Autodesk Fusion 360 part; units mm, degrees
(part 6 of 12)
  arc A2269 (96.3654, -39.4411) -> (96.0604, -39.4411) centre (96.2129, -39.4411) ccw
  arc A2270 (150.9862, -40.1688) -> (151.2912, -40.1688) centre (151.1387, -40.1688) ccw
  arc A2271 (151.2912, -40.1688) -> (150.9862, -40.1688) centre (151.1387, -40.1688) ccw
  arc A2272 (44.7289, -41.9748) -> (45.0339, -41.9748) centre (44.8814, -41.9748) ccw
  arc A2273 (45.0339, -41.9748) -> (44.7289, -41.9748) centre (44.8814, -41.9748) ccw
  arc A2274 (163.9811, 37.8053) -> (164.2861, 37.8053) centre (164.1336, 37.8053) ccw
  arc A2275 (164.2861, 37.8053) -> (163.9811, 37.8053) centre (164.1336, 37.8053) ccw
  arc A2276 (146.0527, -13.2374) -> (146.3577, -13.2374) centre (146.2052, -13.2374) ccw
  arc A2277 (146.3577, -13.2374) -> (146.0527, -13.2374) centre (146.2052, -13.2374) ccw
  arc A2278 (176.4441, -9.8328) -> (176.7491, -9.8328) centre (176.5966, -9.8328) ccw
  arc A2279 (176.7491, -9.8328) -> (176.4441, -9.8328) centre (176.5966, -9.8328) ccw
  arc A2280 (116.1959, -12.0024) -> (115.8909, -12.0024) centre (116.0434, -12.0024) ccw
  arc A2281 (115.8909, -12.0024) -> (116.1959, -12.0024) centre (116.0434, -12.0024) ccw
  arc A2282 (150.7728, -10.1653) -> (150.4678, -10.1653) centre (150.6203, -10.1653) ccw
  arc A2283 (150.4678, -10.1653) -> (150.7728, -10.1653) centre (150.6203, -10.1653) ccw
  arc A2284 (85.9928, -12.5211) -> (86.2978, -12.5211) centre (86.1453, -12.5211) ccw
  arc A2285 (86.2978, -12.5211) -> (85.9928, -12.5211) centre (86.1453, -12.5211) ccw
  arc A2286 (116.6014, -9.5793) -> (116.9064, -9.5793) centre (116.7539, -9.5793) ccw
  arc A2287 (116.9064, -9.5793) -> (116.6014, -9.5793) centre (116.7539, -9.5793) ccw
  arc A2288 (43.8853, -19.9798) -> (44.1903, -19.9798) centre (44.0378, -19.9798) ccw
  arc A2289 (44.1903, -19.9798) -> (43.8853, -19.9798) centre (44.0378, -19.9798) ccw
  arc A2290 (91.0235, -13.194) -> (91.3285, -13.194) centre (91.176, -13.194) ccw
  arc A2291 (91.3285, -13.194) -> (91.0235, -13.194) centre (91.176, -13.194) ccw
  arc A2292 (217.3525, -62.0055) -> (217.6575, -62.0055) centre (217.505, -62.0055) ccw
  arc A2293 (217.6575, -62.0055) -> (217.3525, -62.0055) centre (217.505, -62.0055) ccw
  arc A2294 (186.1886, -6.5094) -> (185.8836, -6.5094) centre (186.0361, -6.5094) ccw
  arc A2295 (185.8836, -6.5094) -> (186.1886, -6.5094) centre (186.0361, -6.5094) ccw
  arc A2296 (150.3339, -28.8564) -> (150.6389, -28.8564) centre (150.4864, -28.8564) ccw
  arc A2297 (150.6389, -28.8564) -> (150.3339, -28.8564) centre (150.4864, -28.8564) ccw
  arc A2298 (145.1401, -60.2572) -> (145.4451, -60.2572) centre (145.2926, -60.2572) ccw
  arc A2299 (145.4451, -60.2572) -> (145.1401, -60.2572) centre (145.2926, -60.2572) ccw
  arc A2300 (119.5917, -66.7802) -> (119.8967, -66.7802) centre (119.7442, -66.7802) ccw
  arc A2301 (119.8967, -66.7802) -> (119.5917, -66.7802) centre (119.7442, -66.7802) ccw
  arc A2302 (168.2221, 11.5998) -> (168.5272, 11.5998) centre (168.3747, 11.5998) ccw
  arc A2303 (168.5272, 11.5998) -> (168.2221, 11.5998) centre (168.3747, 11.5998) ccw
  arc A2304 (194.7456, 20.9148) -> (195.0506, 20.9148) centre (194.8981, 20.9148) ccw
  arc A2305 (195.0506, 20.9148) -> (194.7456, 20.9148) centre (194.8981, 20.9148) ccw
  arc A2306 (99.0245, 26.218) -> (99.3295, 26.218) centre (99.177, 26.218) ccw
  arc A2307 (99.3295, 26.218) -> (99.0245, 26.218) centre (99.177, 26.218) ccw
  arc A2308 (70.4291, -16.6778) -> (70.1241, -16.6778) centre (70.2766, -16.6778) ccw
  arc A2309 (70.1241, -16.6778) -> (70.4291, -16.6778) centre (70.2766, -16.6778) ccw
  arc A2310 (134.9499, 16.8688) -> (135.2549, 16.8688) centre (135.1024, 16.8688) ccw
  arc A2311 (135.2549, 16.8688) -> (134.9499, 16.8688) centre (135.1024, 16.8688) ccw
  arc A2312 (165.5168, 20.1454) -> (165.8218, 20.1454) centre (165.6693, 20.1454) ccw
  arc A2313 (165.8218, 20.1454) -> (165.5168, 20.1454) centre (165.6693, 20.1454) ccw
  arc A2314 (100.893, 26.9607) -> (101.198, 26.9607) centre (101.0455, 26.9607) ccw
  arc A2315 (101.198, 26.9607) -> (100.893, 26.9607) centre (101.0455, 26.9607) ccw
  arc A2316 (86.6801, -6.1922) -> (86.9851, -6.1922) centre (86.8326, -6.1922) ccw
  arc A2317 (86.9851, -6.1922) -> (86.6801, -6.1922) centre (86.8326, -6.1922) ccw
  arc A2318 (104.3532, 16.8617) -> (104.6582, 16.8617) centre (104.5057, 16.8617) ccw
  arc A2319 (104.6582, 16.8617) -> (104.3532, 16.8617) centre (104.5057, 16.8617) ccw
  arc A2320 (124.5234, 15.4924) -> (124.8284, 15.4924) centre (124.6759, 15.4924) ccw
  arc A2321 (124.8284, 15.4924) -> (124.5234, 15.4924) centre (124.6759, 15.4924) ccw
  arc A2322 (20.8272, 14.645) -> (21.1322, 14.645) centre (20.9797, 14.645) ccw
  arc A2323 (21.1322, 14.645) -> (20.8272, 14.645) centre (20.9797, 14.645) ccw
  arc A2324 (21.2366, 18.769) -> (21.5416, 18.769) centre (21.3891, 18.769) ccw
  arc A2325 (21.5416, 18.769) -> (21.2366, 18.769) centre (21.3891, 18.769) ccw
  arc A2326 (38.9043, 16.8274) -> (38.5993, 16.8274) centre (38.7518, 16.8274) ccw
  arc A2327 (38.5993, 16.8274) -> (38.9043, 16.8274) centre (38.7518, 16.8274) ccw
  arc A2328 (75.6966, 20.0435) -> (76.0016, 20.0435) centre (75.8491, 20.0435) ccw
  arc A2329 (76.0016, 20.0435) -> (75.6966, 20.0435) centre (75.8491, 20.0435) ccw
  arc A2330 (216.5973, 36.5028) -> (216.9023, 36.5028) centre (216.7498, 36.5028) ccw
  arc A2331 (216.9023, 36.5028) -> (216.5973, 36.5028) centre (216.7498, 36.5028) ccw
  arc A2332 (62.4485, 36.5028) -> (62.7535, 36.5028) centre (62.601, 36.5028) ccw
  arc A2333 (62.7535, 36.5028) -> (62.4485, 36.5028) centre (62.601, 36.5028) ccw
  arc A2334 (124.4947, 49.6851) -> (124.7997, 49.6851) centre (124.6472, 49.6851) ccw
  arc A2335 (124.7997, 49.6851) -> (124.4947, 49.6851) centre (124.6472, 49.6851) ccw
  arc A2336 (92.9478, -27.5572) -> (93.2528, -27.5572) centre (93.1003, -27.5572) ccw
  arc A2337 (93.2528, -27.5572) -> (92.9478, -27.5572) centre (93.1003, -27.5572) ccw
  arc A2338 (158.911, 44.4614) -> (159.216, 44.4614) centre (159.0635, 44.4614) ccw
  arc A2339 (159.216, 44.4614) -> (158.911, 44.4614) centre (159.0635, 44.4614) ccw
  arc A2340 (184.7538, 44.4614) -> (185.0588, 44.4614) centre (184.9063, 44.4614) ccw
  arc A2341 (185.0588, 44.4614) -> (184.7538, 44.4614) centre (184.9063, 44.4614) ccw
  arc A2342 (118.6672, 12.5444) -> (118.9722, 12.5444) centre (118.8197, 12.5444) ccw
  arc A2343 (118.9722, 12.5444) -> (118.6672, 12.5444) centre (118.8197, 12.5444) ccw
  arc A2344 (127.2216, 57.1512) -> (127.5266, 57.1512) centre (127.3741, 57.1512) ccw
  arc A2345 (127.5266, 57.1512) -> (127.2216, 57.1512) centre (127.3741, 57.1512) ccw
  arc A2346 (128.9905, 44.4614) -> (129.2955, 44.4614) centre (129.143, 44.4614) ccw
  arc A2347 (129.2955, 44.4614) -> (128.9905, 44.4614) centre (129.143, 44.4614) ccw
  arc A2348 (159.434, 50.1576) -> (159.739, 50.1576) centre (159.5865, 50.1576) ccw
  arc A2349 (159.739, 50.1576) -> (159.434, 50.1576) centre (159.5865, 50.1576) ccw
  arc A2350 (98.9415, 44.4614) -> (99.2465, 44.4614) centre (99.094, 44.4614) ccw
  arc A2351 (99.2465, 44.4614) -> (98.9415, 44.4614) centre (99.094, 44.4614) ccw
  arc A2352 (106.8124, 44.4614) -> (107.1174, 44.4614) centre (106.9649, 44.4614) ccw
  arc A2353 (107.1174, 44.4614) -> (106.8124, 44.4614) centre (106.9649, 44.4614) ccw
  arc A2354 (112.9504, 50.5993) -> (113.2554, 50.5993) centre (113.1029, 50.5993) ccw
  arc A2355 (113.2554, 50.5993) -> (112.9504, 50.5993) centre (113.1029, 50.5993) ccw
  arc A2356 (129.2079, 50.5993) -> (129.5129, 50.5993) centre (129.3604, 50.5993) ccw
  arc A2357 (129.5129, 50.5993) -> (129.2079, 50.5993) centre (129.3604, 50.5993) ccw
  arc A2358 (68.8676, 44.4614) -> (69.1726, 44.4614) centre (69.0201, 44.4614) ccw
  arc A2359 (69.1726, 44.4614) -> (68.8676, 44.4614) centre (69.0201, 44.4614) ccw
  arc A2360 (99.6842, 49.9803) -> (99.9892, 49.9803) centre (99.8367, 49.9803) ccw
  arc A2361 (99.9892, 49.9803) -> (99.6842, 49.9803) centre (99.8367, 49.9803) ccw
  arc A2362 (51.0316, 50.5033) -> (51.3367, 50.5033) centre (51.1842, 50.5033) ccw
  arc A2363 (51.3367, 50.5033) -> (51.0316, 50.5033) centre (51.1842, 50.5033) ccw
  arc A2364 (73.5005, 49.883) -> (73.8055, 49.883) centre (73.653, 49.883) ccw
  arc A2365 (73.8055, 49.883) -> (73.5005, 49.883) centre (73.653, 49.883) ccw
  arc A2366 (221.1025, -27.0019) -> (221.4075, -27.0019) centre (221.255, -27.0019) ccw
  arc A2367 (221.4075, -27.0019) -> (221.1025, -27.0019) centre (221.255, -27.0019) ccw
  arc A2368 (218.1536, 60.5599) -> (218.4586, 60.5599) centre (218.3061, 60.5599) ccw
  arc A2369 (218.4586, 60.5599) -> (218.1536, 60.5599) centre (218.3061, 60.5599) ccw
  arc A2370 (43.6496, 60.5599) -> (43.9546, 60.5599) centre (43.8021, 60.5599) ccw
  arc A2371 (43.9546, 60.5599) -> (43.6496, 60.5599) centre (43.8021, 60.5599) ccw
  arc A2372 (188.8485, 74.8421) -> (189.1535, 74.8421) centre (189.001, 74.8421) ccw
  arc A2373 (189.1535, 74.8421) -> (188.8485, 74.8421) centre (189.001, 74.8421) ccw
  arc A2374 (200.9369, 74.8421) -> (201.2419, 74.8421) centre (201.0894, 74.8421) ccw
  arc A2375 (201.2419, 74.8421) -> (200.9369, 74.8421) centre (201.0894, 74.8421) ccw
  arc A2376 (95.5287, 66.3102) -> (95.2237, 66.3102) centre (95.3762, 66.3102) ccw
  arc A2377 (95.2237, 66.3102) -> (95.5287, 66.3102) centre (95.3762, 66.3102) ccw
  arc A2378 (63.9466, -23.0278) -> (64.2516, -23.0278) centre (64.0991, -23.0278) ccw
  arc A2379 (64.2516, -23.0278) -> (63.9466, -23.0278) centre (64.0991, -23.0278) ccw
  arc A2380 (92.0195, -20.5656) -> (92.3245, -20.5656) centre (92.172, -20.5656) ccw
  arc A2381 (92.3245, -20.5656) -> (92.0195, -20.5656) centre (92.172, -20.5656) ccw
  arc A2382 (65.5109, 83.9028) -> (65.816, 83.9028) centre (65.6634, 83.9028) ccw
  arc A2383 (65.816, 83.9028) -> (65.5109, 83.9028) centre (65.6634, 83.9028) ccw
  arc A2384 (35.4591, -9.865) -> (35.7641, -9.865) centre (35.6116, -9.865) ccw
  arc A2385 (35.7641, -9.865) -> (35.4591, -9.865) centre (35.6116, -9.865) ccw
  arc A2386 (35.4568, -3.5704) -> (35.7618, -3.5704) centre (35.6093, -3.5704) ccw
  arc A2387 (35.7618, -3.5704) -> (35.4568, -3.5704) centre (35.6093, -3.5704) ccw
  arc A2388 (69.1045, 74.231) -> (69.4096, 74.231) centre (69.257, 74.231) ccw
  arc A2389 (69.4096, 74.231) -> (69.1045, 74.231) centre (69.257, 74.231) ccw
  arc A2390 (104.9132, 74.231) -> (104.6082, 74.231) centre (104.7607, 74.231) ccw
  arc A2391 (104.6082, 74.231) -> (104.9132, 74.231) centre (104.7607, 74.231) ccw
  arc A2392 (18.7687, -49.6804) -> (18.4637, -49.6804) centre (18.6162, -49.6804) ccw
  arc A2393 (18.4637, -49.6804) -> (18.7687, -49.6804) centre (18.6162, -49.6804) ccw
  arc A2394 (22.6862, -60.4264) -> (22.3812, -60.4264) centre (22.5337, -60.4264) ccw
  arc A2395 (22.3812, -60.4264) -> (22.6862, -60.4264) centre (22.5337, -60.4264) ccw
  arc A2396 (142.6481, 77.1248) -> (142.3431, 77.1248) centre (142.4956, 77.1248) ccw
  arc A2397 (142.3431, 77.1248) -> (142.6481, 77.1248) centre (142.4956, 77.1248) ccw
  arc A2398 (134.7352, 77.1248) -> (134.4302, 77.1248) centre (134.5827, 77.1248) ccw
  arc A2399 (134.4302, 77.1248) -> (134.7352, 77.1248) centre (134.5827, 77.1248) ccw
  arc A2400 (155.7745, 57.7646) -> (155.4695, 57.7646) centre (155.622, 57.7646) ccw
  arc A2401 (155.4695, 57.7646) -> (155.7745, 57.7646) centre (155.622, 57.7646) ccw
  arc A2402 (159.8904, 57.7646) -> (159.5854, 57.7646) centre (159.7379, 57.7646) ccw
  arc A2403 (159.5854, 57.7646) -> (159.8904, 57.7646) centre (159.7379, 57.7646) ccw
  arc A2404 (5.7362, 29.8711) -> (5.4312, 29.8711) centre (5.5837, 29.8711) ccw
  arc A2405 (5.4312, 29.8711) -> (5.7362, 29.8711) centre (5.5837, 29.8711) ccw
  arc A2406 (13.8419, -37.0289) -> (13.5369, -37.0289) centre (13.6894, -37.0289) ccw
  arc A2407 (13.5369, -37.0289) -> (13.8419, -37.0289) centre (13.6894, -37.0289) ccw
  arc A2408 (13.0738, -57.8284) -> (12.7688, -57.8284) centre (12.9213, -57.8284) ccw
  arc A2409 (12.7688, -57.8284) -> (13.0738, -57.8284) centre (12.9213, -57.8284) ccw
  arc A2410 (16.8027, -57.3339) -> (16.4977, -57.3339) centre (16.6502, -57.3339) ccw
  arc A2411 (16.4977, -57.3339) -> (16.8027, -57.3339) centre (16.6502, -57.3339) ccw
  arc A2412 (10.6361, 67.0153) -> (10.3311, 67.0153) centre (10.4836, 67.0153) ccw
  arc A2413 (10.3311, 67.0153) -> (10.6361, 67.0153) centre (10.4836, 67.0153) ccw
  arc A2414 (14.7771, 16.4842) -> (14.4721, 16.4842) centre (14.6246, 16.4842) ccw
  arc A2415 (14.4721, 16.4842) -> (14.7771, 16.4842) centre (14.6246, 16.4842) ccw
  arc A2416 (23.579, 16.4842) -> (23.274, 16.4842) centre (23.4265, 16.4842) ccw
  arc A2417 (23.274, 16.4842) -> (23.579, 16.4842) centre (23.4265, 16.4842) ccw
  arc A2418 (17.122, -56.3786) -> (16.817, -56.3786) centre (16.9695, -56.3786) ccw
  arc A2419 (16.817, -56.3786) -> (17.122, -56.3786) centre (16.9695, -56.3786) ccw
  arc A2420 (15.17, -53.6621) -> (14.865, -53.6621) centre (15.0175, -53.6621) ccw
  arc A2421 (14.865, -53.6621) -> (15.17, -53.6621) centre (15.0175, -53.6621) ccw
  arc A2422 (16.2236, -61.0169) -> (15.9186, -61.0169) centre (16.0711, -61.0169) ccw
  arc A2423 (15.9186, -61.0169) -> (16.2236, -61.0169) centre (16.0711, -61.0169) ccw
  arc A2424 (161.3656, -5.432) -> (161.0606, -5.432) centre (161.2131, -5.432) ccw
  arc A2425 (161.0606, -5.432) -> (161.3656, -5.432) centre (161.2131, -5.432) ccw
  arc A2426 (41.9593, -4.8617) -> (42.2643, -4.8617) centre (42.1118, -4.8617) ccw
  arc A2427 (42.2643, -4.8617) -> (41.9593, -4.8617) centre (42.1118, -4.8617) ccw
  arc A2428 (217.7147, 48.9513) -> (218.0197, 48.9513) centre (217.8672, 48.9513) ccw
  arc A2429 (218.0197, 48.9513) -> (217.7147, 48.9513) centre (217.8672, 48.9513) ccw
  arc A2430 (192.6885, -2.8919) -> (192.9935, -2.8919) centre (192.841, -2.8919) ccw
  arc A2431 (192.9935, -2.8919) -> (192.6885, -2.8919) centre (192.841, -2.8919) ccw
  arc A2432 (208.6974, 31.9866) -> (209.0024, 31.9866) centre (208.8499, 31.9866) ccw
  arc A2433 (209.0024, 31.9866) -> (208.6974, 31.9866) centre (208.8499, 31.9866) ccw
  arc A2434 (186.4678, 14.4761) -> (186.7728, 14.4761) centre (186.6203, 14.4761) ccw
  arc A2435 (186.7728, 14.4761) -> (186.4678, 14.4761) centre (186.6203, 14.4761) ccw
  arc A2436 (195.5797, 7.3252) -> (195.2747, 7.3252) centre (195.4272, 7.3252) ccw
  arc A2437 (195.2747, 7.3252) -> (195.5797, 7.3252) centre (195.4272, 7.3252) ccw
  arc A2438 (12.9115, -60.0847) -> (13.2165, -60.0847) centre (13.064, -60.0847) ccw
  arc A2439 (13.2165, -60.0847) -> (12.9115, -60.0847) centre (13.064, -60.0847) ccw
  arc A2440 (11.0604, 12.8002) -> (11.3654, 12.8002) centre (11.2129, 12.8002) ccw
  arc A2441 (11.3654, 12.8002) -> (11.0604, 12.8002) centre (11.2129, 12.8002) ccw
  arc A2442 (9.4177, 70.1903) -> (9.7227, 70.1903) centre (9.5702, 70.1903) ccw
  arc A2443 (9.7227, 70.1903) -> (9.4177, 70.1903) centre (9.5702, 70.1903) ccw
  arc A2444 (188.0484, 15.9968) -> (188.3534, 15.9968) centre (188.2009, 15.9968) ccw
  arc A2445 (188.3534, 15.9968) -> (188.0484, 15.9968) centre (188.2009, 15.9968) ccw
  arc A2446 (194.8569, 9.8652) -> (195.1619, 9.8652) centre (195.0094, 9.8652) ccw
  arc A2447 (195.1619, 9.8652) -> (194.8569, 9.8652) centre (195.0094, 9.8652) ccw
  arc A2448 (37.3095, 59.1472) -> (37.6145, 59.1472) centre (37.462, 59.1472) ccw
  arc A2449 (37.6145, 59.1472) -> (37.3095, 59.1472) centre (37.462, 59.1472) ccw
  arc A2450 (172.1022, 3.3052) -> (171.7972, 3.3052) centre (171.9497, 3.3052) ccw
  arc A2451 (171.7972, 3.3052) -> (172.1022, 3.3052) centre (171.9497, 3.3052) ccw
  arc A2452 (19.8073, 20.1403) -> (19.5023, 20.1403) centre (19.6548, 20.1403) ccw
  arc A2453 (19.5023, 20.1403) -> (19.8073, 20.1403) centre (19.6548, 20.1403) ccw
  arc A2454 (196.5335, 32.2079) -> (196.2285, 32.2079) centre (196.381, 32.2079) ccw
  arc A2455 (196.2285, 32.2079) -> (196.5335, 32.2079) centre (196.381, 32.2079) ccw
  arc A2456 (65.4614, -31.7901) -> (65.7664, -31.7901) centre (65.6139, -31.7901) ccw
  arc A2457 (65.7664, -31.7901) -> (65.4614, -31.7901) centre (65.6139, -31.7901) ccw
  arc A2458 (99.6562, 28.1421) -> (99.9612, 28.1421) centre (99.8087, 28.1421) ccw
  arc A2459 (99.9612, 28.1421) -> (99.6562, 28.1421) centre (99.8087, 28.1421) ccw
  arc A2460 (38.9151, 74.6874) -> (39.2201, 74.6874) centre (39.0676, 74.6874) ccw
  arc A2461 (39.2201, 74.6874) -> (38.9151, 74.6874) centre (39.0676, 74.6874) ccw
  arc A2462 (68.325, 81.757) -> (68.63, 81.757) centre (68.4775, 81.757) ccw
  arc A2463 (68.63, 81.757) -> (68.325, 81.757) centre (68.4775, 81.757) ccw
  arc A2464 (98.9636, 74.853) -> (99.2686, 74.853) centre (99.1161, 74.853) ccw
  arc A2465 (99.2686, 74.853) -> (98.9636, 74.853) centre (99.1161, 74.853) ccw
  arc A2466 (129.4358, 80.5774) -> (129.7408, 80.5774) centre (129.5883, 80.5774) ccw
  arc A2467 (129.7408, 80.5774) -> (129.4358, 80.5774) centre (129.5883, 80.5774) ccw
  arc A2468 (159.1353, 74.2089) -> (159.4403, 74.2089) centre (159.2878, 74.2089) ccw
  arc A2469 (159.4403, 74.2089) -> (159.1353, 74.2089) centre (159.2878, 74.2089) ccw
  arc A2470 (194.3174, 74.2089) -> (194.6224, 74.2089) centre (194.4699, 74.2089) ccw
  arc A2471 (194.6224, 74.2089) -> (194.3174, 74.2089) centre (194.4699, 74.2089) ccw
  arc A2472 (191.848, 42.1421) -> (192.153, 42.1421) centre (192.0005, 42.1421) ccw
  arc A2473 (192.153, 42.1421) -> (191.848, 42.1421) centre (192.0005, 42.1421) ccw
  arc A2474 (215.2414, 42.1421) -> (214.9364, 42.1421) centre (215.0889, 42.1421) ccw
  arc A2475 (214.9364, 42.1421) -> (215.2414, 42.1421) centre (215.0889, 42.1421) ccw
  arc A2476 (74.0609, 16.8462) -> (74.3659, 16.8462) centre (74.2134, 16.8462) ccw
  arc A2477 (74.3659, 16.8462) -> (74.0609, 16.8462) centre (74.2134, 16.8462) ccw
  arc A2478 (109.5709, 19.9249) -> (109.8759, 19.9249) centre (109.7234, 19.9249) ccw
  arc A2479 (109.8759, 19.9249) -> (109.5709, 19.9249) centre (109.7234, 19.9249) ccw
  arc A2480 (180.3037, -15.9405) -> (180.6087, -15.9405) centre (180.4562, -15.9405) ccw
  arc A2481 (180.6087, -15.9405) -> (180.3037, -15.9405) centre (180.4562, -15.9405) ccw
  arc A2482 (206.7964, -9.7413) -> (207.1014, -9.7413) centre (206.9489, -9.7413) ccw
  arc A2483 (207.1014, -9.7413) -> (206.7964, -9.7413) centre (206.9489, -9.7413) ccw
  arc A2484 (101.0151, -25.7268) -> (101.3201, -25.7268) centre (101.1676, -25.7268) ccw
  arc A2485 (101.3201, -25.7268) -> (101.0151, -25.7268) centre (101.1676, -25.7268) ccw
extrude "Extrude1" add sketch "PCB_LEFT_MAIN" along normal blind 1.5 contours L0 L1 L2 L3 L4 L5 L6 L7 L8 L9 L10 L11 L12 L13 L14 L15 L16 L17 L18 L564 makes body 1
sketch "PCB_RIGHT_MAIN" plane through (0, 0, 0) normal (0, 0, 1) x (1, 0, 0)
  line L0 (-214.2494, -136.0173) -> (90.1702, -136.0173)
  line L1 (90.1702, 37.2111) -> (-197.4854, 37.2111)
  line L2 (90.1702, -136.0173) -> (90.1702, 37.2111)
  line L3 (-214.1224, -136.0173) -> (-214.2494, -136.0173)
  line L4 (-214.2494, -136.0173) -> (-214.2494, -123.6982)
  line L5 (-208.6614, -17.907) -> (-204.5974, -17.907)
  line L6 (-198.5014, -107.9502) -> (-198.5014, -82.9312)
  line L7 (-214.2494, -123.6982) -> (-198.5014, -107.9502)
  line L8 (-198.5014, -82.9312) -> (-199.5174, -82.9312)
  line L9 (-199.5174, -82.9312) -> (-208.6614, -73.7871)
  line L10 (-208.6614, -73.7871) -> (-208.6614, -17.907)
  line L11 (-204.5974, -17.907) -> (-197.4854, -10.795)
  line L12 (-197.4854, -10.795) -> (-197.4854, 37.2111)
  line L13 (80.7041, -119.8472) -> (81.6042, -119.8472)
  line L14 (80.7041, -111.5472) -> (81.6042, -111.5472)
  line L15 (80.7041, -118.7473) -> (80.7041, -119.8472)
  line L16 (80.7041, -112.6473) -> (80.7041, -111.5472)
  line L17 (81.4143, -112.6473) -> (80.7041, -112.6473)
  line L18 (80.7041, -118.7473) -> (81.3296, -118.7473)
  line L19 (81.3296, -118.7473) -> (81.3482, -118.7473)
  arc A0 (81.3482, -118.7473) -> (81.6041, -118.4913) centre (81.3481, -118.4912) ccw
  line L20 (81.6041, -118.4383) -> (81.6041, -112.8371)
  arc A1 (81.6041, -112.8371) -> (81.4143, -112.6473) centre (81.4142, -112.8372) ccw
  arc A2 (80.7041, -119.6343) -> (80.7062, -119.6322) centre (80.7062, -119.6343) cw
  line L21 (80.7041, -119.8472) -> (81.6042, -119.8472)
  line L22 (80.7041, -111.5472) -> (81.6042, -111.5472)
  line L23 (80.7041, -118.7473) -> (80.7041, -119.8472)
  line L24 (80.7041, -112.6473) -> (80.7041, -111.5472)
  line L25 (81.4143, -112.6473) -> (80.7041, -112.6473)
  line L26 (80.7041, -118.7473) -> (81.3296, -118.7473)
  line L27 (81.3296, -118.7473) -> (81.3482, -118.7473)
  arc A3 (81.3482, -118.7473) -> (81.6041, -118.4913) centre (81.3481, -118.4912) ccw
  line L28 (81.6041, -118.4383) -> (81.6041, -112.8371)
  arc A4 (81.6041, -112.8371) -> (81.4143, -112.6473) centre (81.4142, -112.8372) ccw
  arc A5 (80.7041, -119.6343) -> (80.7062, -119.6322) centre (80.7062, -119.6343) cw
  arc A6 (-180.5461, 25.047) -> (-184.5339, 25.047) centre (-182.54, 25.047) ccw
  arc A7 (-184.5339, 25.047) -> (-180.5461, 25.047) centre (-182.54, 25.047) ccw
  arc A8 (-178.3109, 24.92) -> (-176.6091, 24.92) centre (-177.46, 24.92) ccw
  arc A9 (-176.6091, 24.92) -> (-178.3109, 24.92) centre (-177.46, 24.92) ccw
  arc A10 (-188.4709, 24.92) -> (-186.7691, 24.92) centre (-187.62, 24.92) ccw
  arc A11 (-186.7691, 24.92) -> (-188.4709, 24.92) centre (-187.62, 24.92) ccw
  arc A12 (-154.5339, 25.047) -> (-150.5461, 25.047) centre (-152.54, 25.047) ccw
  arc A13 (-150.5461, 25.047) -> (-154.5339, 25.047) centre (-152.54, 25.047) ccw
  arc A14 (-146.6091, 24.92) -> (-148.3109, 24.92) centre (-147.46, 24.92) ccw
  arc A15 (-148.3109, 24.92) -> (-146.6091, 24.92) centre (-147.46, 24.92) ccw
  arc A16 (-156.7691, 24.92) -> (-158.4709, 24.92) centre (-157.62, 24.92) ccw
  arc A17 (-158.4709, 24.92) -> (-156.7691, 24.92) centre (-157.62, 24.92) ccw
  arc A18 (-120.5461, 25.047) -> (-124.5339, 25.047) centre (-122.54, 25.047) ccw
  arc A19 (-124.5339, 25.047) -> (-120.5461, 25.047) centre (-122.54, 25.047) ccw
  arc A20 (-118.3109, 24.92) -> (-116.6091, 24.92) centre (-117.46, 24.92) ccw
  arc A21 (-116.6091, 24.92) -> (-118.3109, 24.92) centre (-117.46, 24.92) ccw
  arc A22 (-128.4709, 24.92) -> (-126.7691, 24.92) centre (-127.62, 24.92) ccw
  arc A23 (-126.7691, 24.92) -> (-128.4709, 24.92) centre (-127.62, 24.92) ccw
  arc A24 (-94.5339, 25.047) -> (-90.5461, 25.047) centre (-92.54, 25.047) ccw
  arc A25 (-90.5461, 25.047) -> (-94.5339, 25.047) centre (-92.54, 25.047) ccw
  arc A26 (-86.6091, 24.92) -> (-88.3109, 24.92) centre (-87.46, 24.92) ccw
  arc A27 (-88.3109, 24.92) -> (-86.6091, 24.92) centre (-87.46, 24.92) ccw
  arc A28 (-98.4709, 24.92) -> (-96.7691, 24.92) centre (-97.62, 24.92) ccw
  arc A29 (-96.7691, 24.92) -> (-98.4709, 24.92) centre (-97.62, 24.92) ccw
  arc A30 (-64.5339, 25.047) -> (-60.5461, 25.047) centre (-62.54, 25.047) ccw
  arc A31 (-60.5461, 25.047) -> (-64.5339, 25.047) centre (-62.54, 25.047) ccw
  arc A32 (-58.3109, 24.92) -> (-56.6091, 24.92) centre (-57.46, 24.92) ccw
  arc A33 (-56.6091, 24.92) -> (-58.3109, 24.92) centre (-57.46, 24.92) ccw
  arc A34 (-66.7691, 24.92) -> (-68.4709, 24.92) centre (-67.62, 24.92) ccw
  arc A35 (-68.4709, 24.92) -> (-66.7691, 24.92) centre (-67.62, 24.92) ccw
  arc A36 (-34.5339, 25.047) -> (-30.5461, 25.047) centre (-32.54, 25.047) ccw
  arc A37 (-30.5461, 25.047) -> (-34.5339, 25.047) centre (-32.54, 25.047) ccw
  arc A38 (-28.3109, 24.92) -> (-26.6091, 24.92) centre (-27.46, 24.92) ccw
  arc A39 (-26.6091, 24.92) -> (-28.3109, 24.92) centre (-27.46, 24.92) ccw
  arc A40 (-38.4709, 24.92) -> (-36.7691, 24.92) centre (-37.62, 24.92) ccw
  arc A41 (-36.7691, 24.92) -> (-38.4709, 24.92) centre (-37.62, 24.92) ccw
  arc A42 (-0.5461, 25.047) -> (-4.5339, 25.047) centre (-2.54, 25.047) ccw
  arc A43 (-4.5339, 25.047) -> (-0.5461, 25.047) centre (-2.54, 25.047) ccw
  arc A44 (1.6891, 24.92) -> (3.3909, 24.92) centre (2.54, 24.92) ccw
  arc A45 (3.3909, 24.92) -> (1.6891, 24.92) centre (2.54, 24.92) ccw
  arc A46 (-6.7691, 24.92) -> (-8.4709, 24.92) centre (-7.62, 24.92) ccw
  arc A47 (-8.4709, 24.92) -> (-6.7691, 24.92) centre (-7.62, 24.92) ccw
  arc A48 (25.4661, 25.047) -> (29.4539, 25.047) centre (27.46, 25.047) ccw
  arc A49 (29.4539, 25.047) -> (25.4661, 25.047) centre (27.46, 25.047) ccw
  arc A50 (33.3909, 24.92) -> (31.6891, 24.92) centre (32.54, 24.92) ccw
  arc A51 (31.6891, 24.92) -> (33.3909, 24.92) centre (32.54, 24.92) ccw
  arc A52 (23.2309, 24.92) -> (21.5291, 24.92) centre (22.38, 24.92) ccw
  arc A53 (21.5291, 24.92) -> (23.2309, 24.92) centre (22.38, 24.92) ccw
  arc A54 (-184.5339, -4.953) -> (-180.5461, -4.953) centre (-182.54, -4.953) ccw
  arc A55 (-180.5461, -4.953) -> (-184.5339, -4.953) centre (-182.54, -4.953) ccw
  arc A56 (-176.6091, -5.08) -> (-178.3109, -5.08) centre (-177.46, -5.08) ccw
  arc A57 (-178.3109, -5.08) -> (-176.6091, -5.08) centre (-177.46, -5.08) ccw
  arc A58 (-188.4709, -5.08) -> (-186.7691, -5.08) centre (-187.62, -5.08) ccw
  arc A59 (-186.7691, -5.08) -> (-188.4709, -5.08) centre (-187.62, -5.08) ccw
  arc A60 (-154.5339, -4.953) -> (-150.5461, -4.953) centre (-152.54, -4.953) ccw
  arc A61 (-150.5461, -4.953) -> (-154.5339, -4.953) centre (-152.54, -4.953) ccw
  arc A62 (-146.6091, -5.08) -> (-148.3109, -5.08) centre (-147.46, -5.08) ccw
  arc A63 (-148.3109, -5.08) -> (-146.6091, -5.08) centre (-147.46, -5.08) ccw
  arc A64 (-156.7691, -5.08) -> (-158.4709, -5.08) centre (-157.62, -5.08) ccw
  arc A65 (-158.4709, -5.08) -> (-156.7691, -5.08) centre (-157.62, -5.08) ccw
  arc A66 (-124.5339, -4.953) -> (-120.5461, -4.953) centre (-122.54, -4.953) ccw
  arc A67 (-120.5461, -4.953) -> (-124.5339, -4.953) centre (-122.54, -4.953) ccw
  arc A68 (-118.3109, -5.08) -> (-116.6091, -5.08) centre (-117.46, -5.08) ccw
  arc A69 (-116.6091, -5.08) -> (-118.3109, -5.08) centre (-117.46, -5.08) ccw
  arc A70 (-126.7691, -5.08) -> (-128.4709, -5.08) centre (-127.62, -5.08) ccw
  arc A71 (-128.4709, -5.08) -> (-126.7691, -5.08) centre (-127.62, -5.08) ccw
  arc A72 (-94.5339, -4.953) -> (-90.5461, -4.953) centre (-92.54, -4.953) ccw
  arc A73 (-90.5461, -4.953) -> (-94.5339, -4.953) centre (-92.54, -4.953) ccw
  arc A74 (-88.3109, -5.08) -> (-86.6091, -5.08) centre (-87.46, -5.08) ccw
  arc A75 (-86.6091, -5.08) -> (-88.3109, -5.08) centre (-87.46, -5.08) ccw
  arc A76 (-96.7691, -5.08) -> (-98.4709, -5.08) centre (-97.62, -5.08) ccw
  arc A77 (-98.4709, -5.08) -> (-96.7691, -5.08) centre (-97.62, -5.08) ccw
  arc A78 (-60.5461, -4.953) -> (-64.5339, -4.953) centre (-62.54, -4.953) ccw
  arc A79 (-64.5339, -4.953) -> (-60.5461, -4.953) centre (-62.54, -4.953) ccw
  arc A80 (-58.3109, -5.08) -> (-56.6091, -5.08) centre (-57.46, -5.08) ccw
  arc A81 (-56.6091, -5.08) -> (-58.3109, -5.08) centre (-57.46, -5.08) ccw
  arc A82 (-66.7691, -5.08) -> (-68.4709, -5.08) centre (-67.62, -5.08) ccw
  arc A83 (-68.4709, -5.08) -> (-66.7691, -5.08) centre (-67.62, -5.08) ccw
  arc A84 (-34.5339, -4.953) -> (-30.5461, -4.953) centre (-32.54, -4.953) ccw
  arc A85 (-30.5461, -4.953) -> (-34.5339, -4.953) centre (-32.54, -4.953) ccw
  arc A86 (-26.6091, -5.08) -> (-28.3109, -5.08) centre (-27.46, -5.08) ccw
  arc A87 (-28.3109, -5.08) -> (-26.6091, -5.08) centre (-27.46, -5.08) ccw
  arc A88 (-38.4709, -5.08) -> (-36.7691, -5.08) centre (-37.62, -5.08) ccw
  arc A89 (-36.7691, -5.08) -> (-38.4709, -5.08) centre (-37.62, -5.08) ccw
  arc A90 (13.8049, -5.207) -> (9.8171, -5.207) centre (11.811, -5.207) ccw
  arc A91 (9.8171, -5.207) -> (13.8049, -5.207) centre (11.811, -5.207) ccw
  arc A92 (16.0401, -5.334) -> (17.7419, -5.334) centre (16.891, -5.334) ccw
  arc A93 (17.7419, -5.334) -> (16.0401, -5.334) centre (16.891, -5.334) ccw
  arc A94 (7.5819, -5.334) -> (5.8801, -5.334) centre (6.731, -5.334) ccw
  arc A95 (5.8801, -5.334) -> (7.5819, -5.334) centre (6.731, -5.334) ccw
  arc A96 (48.9332, -5.461) -> (52.921, -5.461) centre (50.9271, -5.461) ccw
  arc A97 (52.921, -5.461) -> (48.9332, -5.461) centre (50.9271, -5.461) ccw
  arc A98 (55.1562, -5.588) -> (56.858, -5.588) centre (56.0071, -5.588) ccw
  arc A99 (56.858, -5.588) -> (55.1562, -5.588) centre (56.0071, -5.588) ccw
  arc A100 (46.698, -5.588) -> (44.9962, -5.588) centre (45.8471, -5.588) ccw
  arc A101 (44.9962, -5.588) -> (46.698, -5.588) centre (45.8471, -5.588) ccw
  arc A102 (-192.7661, -33.5281) -> (-196.7539, -33.5281) centre (-194.76, -33.5281) ccw
  arc A103 (-196.7539, -33.5281) -> (-192.7661, -33.5281) centre (-194.76, -33.5281) ccw
  arc A104 (-188.8291, -33.6551) -> (-190.5309, -33.6551) centre (-189.68, -33.6551) ccw
  arc A105 (-190.5309, -33.6551) -> (-188.8291, -33.6551) centre (-189.68, -33.6551) ccw
  arc A106 (-200.6909, -33.6551) -> (-198.9891, -33.6551) centre (-199.84, -33.6551) ccw
  arc A107 (-198.9891, -33.6551) -> (-200.6909, -33.6551) centre (-199.84, -33.6551) ccw
  arc A108 (-162.7661, -33.5281) -> (-166.7539, -33.5281) centre (-164.76, -33.5281) ccw
  arc A109 (-166.7539, -33.5281) -> (-162.7661, -33.5281) centre (-164.76, -33.5281) ccw
  arc A110 (-160.5309, -33.6551) -> (-158.8291, -33.6551) centre (-159.68, -33.6551) ccw
  arc A111 (-158.8291, -33.6551) -> (-160.5309, -33.6551) centre (-159.68, -33.6551) ccw
  arc A112 (-170.6909, -33.6551) -> (-168.9891, -33.6551) centre (-169.84, -33.6551) ccw
  arc A113 (-168.9891, -33.6551) -> (-170.6909, -33.6551) centre (-169.84, -33.6551) ccw
  arc A114 (-136.7539, -33.5281) -> (-132.7661, -33.5281) centre (-134.76, -33.5281) ccw
  arc A115 (-132.7661, -33.5281) -> (-136.7539, -33.5281) centre (-134.76, -33.5281) ccw
  arc A116 (-130.5309, -33.6551) -> (-128.8291, -33.6551) centre (-129.68, -33.6551) ccw
  arc A117 (-128.8291, -33.6551) -> (-130.5309, -33.6551) centre (-129.68, -33.6551) ccw
  arc A118 (-140.6909, -33.6551) -> (-138.9891, -33.6551) centre (-139.84, -33.6551) ccw
  arc A119 (-138.9891, -33.6551) -> (-140.6909, -33.6551) centre (-139.84, -33.6551) ccw
  arc A120 (-106.7539, -33.5281) -> (-102.7661, -33.5281) centre (-104.76, -33.5281) ccw
  arc A121 (-102.7661, -33.5281) -> (-106.7539, -33.5281) centre (-104.76, -33.5281) ccw
  arc A122 (-100.5309, -33.6551) -> (-98.8291, -33.6551) centre (-99.68, -33.6551) ccw
  arc A123 (-98.8291, -33.6551) -> (-100.5309, -33.6551) centre (-99.68, -33.6551) ccw
  arc A124 (-110.6909, -33.6551) -> (-108.9891, -33.6551) centre (-109.84, -33.6551) ccw
  arc A125 (-108.9891, -33.6551) -> (-110.6909, -33.6551) centre (-109.84, -33.6551) ccw
  arc A126 (-72.7661, -33.5281) -> (-76.7539, -33.5281) centre (-74.76, -33.5281) ccw
  arc A127 (-76.7539, -33.5281) -> (-72.7661, -33.5281) centre (-74.76, -33.5281) ccw
  arc A128 (-68.8291, -33.6551) -> (-70.5309, -33.6551) centre (-69.68, -33.6551) ccw
  arc A129 (-70.5309, -33.6551) -> (-68.8291, -33.6551) centre (-69.68, -33.6551) ccw
  arc A130 (-80.6909, -33.6551) -> (-78.9891, -33.6551) centre (-79.84, -33.6551) ccw
  arc A131 (-78.9891, -33.6551) -> (-80.6909, -33.6551) centre (-79.84, -33.6551) ccw
  arc A132 (-42.7661, -33.5281) -> (-46.7539, -33.5281) centre (-44.76, -33.5281) ccw
  arc A133 (-46.7539, -33.5281) -> (-42.7661, -33.5281) centre (-44.76, -33.5281) ccw
  arc A134 (-38.8291, -33.6551) -> (-40.5309, -33.6551) centre (-39.68, -33.6551) ccw
  arc A135 (-40.5309, -33.6551) -> (-38.8291, -33.6551) centre (-39.68, -33.6551) ccw
  arc A136 (-50.6909, -33.6551) -> (-48.9891, -33.6551) centre (-49.84, -33.6551) ccw
  arc A137 (-48.9891, -33.6551) -> (-50.6909, -33.6551) centre (-49.84, -33.6551) ccw
  line L29 (-12.7661, -33.5281) -> (-12.7661, -33.5281)
  arc A138 (-16.7539, -33.5281) -> (-12.7661, -33.5281) centre (-14.76, -33.5281) ccw
  arc A139 (-12.7661, -33.5281) -> (-16.7539, -33.5281) centre (-14.76, -33.5281) ccw
  arc A140 (-10.5309, -33.6551) -> (-8.8291, -33.6551) centre (-9.68, -33.6551) ccw
  arc A141 (-8.8291, -33.6551) -> (-10.5309, -33.6551) centre (-9.68, -33.6551) ccw
  arc A142 (-20.6909, -33.6551) -> (-18.9891, -33.6551) centre (-19.84, -33.6551) ccw
  arc A143 (-18.9891, -33.6551) -> (-20.6909, -33.6551) centre (-19.84, -33.6551) ccw
  arc A144 (17.2339, -33.5281) -> (13.2461, -33.5281) centre (15.24, -33.5281) ccw
  line L30 (17.2339, -33.5281) -> (17.2339, -33.5281)
  arc A145 (13.2461, -33.5281) -> (17.2339, -33.5281) centre (15.24, -33.5281) ccw
  arc A146 (21.1709, -33.6551) -> (19.4691, -33.6551) centre (20.32, -33.6551) ccw
  arc A147 (19.4691, -33.6551) -> (21.1709, -33.6551) centre (20.32, -33.6551) ccw
  arc A148 (9.3091, -33.6551) -> (11.0109, -33.6551) centre (10.16, -33.6551) ccw
  arc A149 (11.0109, -33.6551) -> (9.3091, -33.6551) centre (10.16, -33.6551) ccw
  arc A150 (52.9185, -34.5441) -> (48.9307, -34.5441) centre (50.9246, -34.5441) ccw
  arc A151 (48.9307, -34.5441) -> (52.9185, -34.5441) centre (50.9246, -34.5441) ccw
  arc A152 (55.1537, -34.6711) -> (56.8555, -34.6711) centre (56.0046, -34.6711) ccw
  arc A153 (56.8555, -34.6711) -> (55.1537, -34.6711) centre (56.0046, -34.6711) ccw
  arc A154 (44.9937, -34.6711) -> (46.6955, -34.6711) centre (45.8446, -34.6711) ccw
  arc A155 (46.6955, -34.6711) -> (44.9937, -34.6711) centre (45.8446, -34.6711) ccw
  arc A156 (-189.967, -60.5851) -> (-185.9792, -60.5851) centre (-187.9731, -60.5851) ccw
  arc A157 (-185.9792, -60.5851) -> (-189.967, -60.5851) centre (-187.9731, -60.5851) ccw
  arc A158 (-183.744, -60.7121) -> (-182.0422, -60.7121) centre (-182.8931, -60.7121) ccw
  arc A159 (-182.0422, -60.7121) -> (-183.744, -60.7121) centre (-182.8931, -60.7121) ccw
  arc A160 (-192.2022, -60.7121) -> (-193.904, -60.7121) centre (-193.0531, -60.7121) ccw
  arc A161 (-193.904, -60.7121) -> (-192.2022, -60.7121) centre (-193.0531, -60.7121) ccw
  arc A162 (-159.967, -60.5851) -> (-155.9792, -60.5851) centre (-157.9731, -60.5851) ccw
  arc A163 (-155.9792, -60.5851) -> (-159.967, -60.5851) centre (-157.9731, -60.5851) ccw
  arc A164 (-153.744, -60.7121) -> (-152.0422, -60.7121) centre (-152.8931, -60.7121) ccw
  arc A165 (-152.0422, -60.7121) -> (-153.744, -60.7121) centre (-152.8931, -60.7121) ccw
  arc A166 (-162.2022, -60.7121) -> (-163.904, -60.7121) centre (-163.0531, -60.7121) ccw
  arc A167 (-163.904, -60.7121) -> (-162.2022, -60.7121) centre (-163.0531, -60.7121) ccw
  arc A168 (-125.9792, -60.5851) -> (-129.967, -60.5851) centre (-127.9731, -60.5851) ccw
  arc A169 (-129.967, -60.5851) -> (-125.9792, -60.5851) centre (-127.9731, -60.5851) ccw
  arc A170 (-122.0422, -60.7121) -> (-123.744, -60.7121) centre (-122.8931, -60.7121) ccw
  arc A171 (-123.744, -60.7121) -> (-122.0422, -60.7121) centre (-122.8931, -60.7121) ccw
  arc A172 (-132.2022, -60.7121) -> (-133.904, -60.7121) centre (-133.0531, -60.7121) ccw
  arc A173 (-133.904, -60.7121) -> (-132.2022, -60.7121) centre (-133.0531, -60.7121) ccw
  arc A174 (-99.967, -60.5851) -> (-95.9792, -60.5851) centre (-97.9731, -60.5851) ccw
  arc A175 (-95.9792, -60.5851) -> (-99.967, -60.5851) centre (-97.9731, -60.5851) ccw
  arc A176 (-93.744, -60.7121) -> (-92.0422, -60.7121) centre (-92.8931, -60.7121) ccw
  arc A177 (-92.0422, -60.7121) -> (-93.744, -60.7121) centre (-92.8931, -60.7121) ccw
  arc A178 (-103.904, -60.7121) -> (-102.2022, -60.7121) centre (-103.0531, -60.7121) ccw
  arc A179 (-102.2022, -60.7121) -> (-103.904, -60.7121) centre (-103.0531, -60.7121) ccw
  arc A180 (-69.967, -60.5851) -> (-65.9792, -60.5851) centre (-67.9731, -60.5851) ccw
  arc A181 (-65.9792, -60.5851) -> (-69.967, -60.5851) centre (-67.9731, -60.5851) ccw
  arc A182 (-62.0422, -60.7121) -> (-63.744, -60.7121) centre (-62.8931, -60.7121) ccw
  arc A183 (-63.744, -60.7121) -> (-62.0422, -60.7121) centre (-62.8931, -60.7121) ccw
  arc A184 (-72.2022, -60.7121) -> (-73.904, -60.7121) centre (-73.0531, -60.7121) ccw
  arc A185 (-73.904, -60.7121) -> (-72.2022, -60.7121) centre (-73.0531, -60.7121) ccw
  arc A186 (-35.9792, -60.5851) -> (-39.967, -60.5851) centre (-37.9731, -60.5851) ccw
  arc A187 (-39.967, -60.5851) -> (-35.9792, -60.5851) centre (-37.9731, -60.5851) ccw
  arc A188 (-32.0422, -60.7121) -> (-33.744, -60.7121) centre (-32.8931, -60.7121) ccw
  arc A189 (-33.744, -60.7121) -> (-32.0422, -60.7121) centre (-32.8931, -60.7121) ccw
  arc A190 (-42.2022, -60.7121) -> (-43.904, -60.7121) centre (-43.0531, -60.7121) ccw
  arc A191 (-43.904, -60.7121) -> (-42.2022, -60.7121) centre (-43.0531, -60.7121) ccw
  arc A192 (6.9469, -61.5951) -> (2.9591, -61.5951) centre (4.953, -61.5951) ccw
  arc A193 (2.9591, -61.5951) -> (6.9469, -61.5951) centre (4.953, -61.5951) ccw
  arc A194 (10.8839, -61.7221) -> (9.1821, -61.7221) centre (10.033, -61.7221) ccw
  arc A195 (9.1821, -61.7221) -> (10.8839, -61.7221) centre (10.033, -61.7221) ccw
  arc A196 (-0.9779, -61.7221) -> (0.7239, -61.7221) centre (-0.127, -61.7221) ccw
  arc A197 (0.7239, -61.7221) -> (-0.9779, -61.7221) centre (-0.127, -61.7221) ccw
  arc A198 (-178.7148, -91.6942) -> (-174.7269, -91.6942) centre (-176.7209, -91.6942) ccw
  arc A199 (-174.7269, -91.6942) -> (-178.7148, -91.6942) centre (-176.7209, -91.6942) ccw
  arc A200 (-172.4917, -91.8212) -> (-170.7899, -91.8212) centre (-171.6408, -91.8212) ccw
  arc A201 (-170.7899, -91.8212) -> (-172.4917, -91.8212) centre (-171.6408, -91.8212) ccw
  arc A202 (-180.95, -91.8212) -> (-182.6518, -91.8212) centre (-181.8009, -91.8212) ccw
  arc A203 (-182.6518, -91.8212) -> (-180.95, -91.8212) centre (-181.8009, -91.8212) ccw
  arc A204 (55.842, -68.9611) -> (51.8542, -68.9611) centre (53.8481, -68.9611) ccw
  arc A205 (51.8542, -68.9611) -> (55.842, -68.9611) centre (53.8481, -68.9611) ccw
  arc A206 (58.0772, -69.0881) -> (59.779, -69.0881) centre (58.9281, -69.0881) ccw
  arc A207 (59.779, -69.0881) -> (58.0772, -69.0881) centre (58.9281, -69.0881) ccw
  arc A208 (49.619, -69.0881) -> (47.9172, -69.0881) centre (48.7681, -69.0881) ccw
  arc A209 (47.9172, -69.0881) -> (49.619, -69.0881) centre (48.7681, -69.0881) ccw
  arc A210 (-144.3104, -91.6942) -> (-148.2982, -91.6942) centre (-146.3043, -91.6942) ccw
  arc A211 (-148.2982, -91.6942) -> (-144.3104, -91.6942) centre (-146.3043, -91.6942) ccw
  arc A212 (-140.3734, -91.8212) -> (-142.0752, -91.8212) centre (-141.2243, -91.8212) ccw
  arc A213 (-142.0752, -91.8212) -> (-140.3734, -91.8212) centre (-141.2243, -91.8212) ccw
  arc A214 (-150.5335, -91.8212) -> (-152.2353, -91.8212) centre (-151.3844, -91.8212) ccw
  arc A215 (-152.2353, -91.8212) -> (-150.5335, -91.8212) centre (-151.3844, -91.8212) ccw
  arc A216 (-117.8817, -91.6942) -> (-113.8939, -91.6942) centre (-115.8878, -91.6942) ccw
  arc A217 (-113.8939, -91.6942) -> (-117.8817, -91.6942) centre (-115.8878, -91.6942) ccw
  arc A218 (-109.9569, -91.8212) -> (-111.6587, -91.8212) centre (-110.8078, -91.8212) ccw
  arc A219 (-111.6587, -91.8212) -> (-109.9569, -91.8212) centre (-110.8078, -91.8212) ccw
  arc A220 (-121.8187, -91.8212) -> (-120.1169, -91.8212) centre (-120.9678, -91.8212) ccw
  arc A221 (-120.1169, -91.8212) -> (-121.8187, -91.8212) centre (-120.9678, -91.8212) ccw
  arc A222 (-83.4773, -91.6942) -> (-87.4651, -91.6942) centre (-85.4712, -91.6942) ccw
  arc A223 (-87.4651, -91.6942) -> (-83.4773, -91.6942) centre (-85.4712, -91.6942) ccw
  arc A224 (-79.5403, -91.8212) -> (-81.2421, -91.8212) centre (-80.3912, -91.8212) ccw
  arc A225 (-81.2421, -91.8212) -> (-79.5403, -91.8212) centre (-80.3912, -91.8212) ccw
  arc A226 (-91.4021, -91.8212) -> (-89.7003, -91.8212) centre (-90.5512, -91.8212) ccw
  arc A227 (-89.7003, -91.8212) -> (-91.4021, -91.8212) centre (-90.5512, -91.8212) ccw
  arc A228 (-53.0607, -91.6942) -> (-57.0485, -91.6942) centre (-55.0546, -91.6942) ccw
  arc A229 (-57.0485, -91.6942) -> (-53.0607, -91.6942) centre (-55.0546, -91.6942) ccw
  arc A230 (-50.8255, -91.8212) -> (-49.1237, -91.8212) centre (-49.9746, -91.8212) ccw
  arc A231 (-49.1237, -91.8212) -> (-50.8255, -91.8212) centre (-49.9746, -91.8212) ccw
  arc A232 (-60.9855, -91.8212) -> (-59.2837, -91.8212) centre (-60.1346, -91.8212) ccw
  arc A233 (-59.2837, -91.8212) -> (-60.9855, -91.8212) centre (-60.1346, -91.8212) ccw
  arc A234 (-22.6441, -91.6942) -> (-26.632, -91.6942) centre (-24.638, -91.6942) ccw
  arc A235 (-26.632, -91.6942) -> (-22.6441, -91.6942) centre (-24.638, -91.6942) ccw
  arc A236 (-18.7071, -91.8212) -> (-20.4089, -91.8212) centre (-19.558, -91.8212) ccw
  arc A237 (-20.4089, -91.8212) -> (-18.7071, -91.8212) centre (-19.558, -91.8212) ccw
  arc A238 (-28.8672, -91.8212) -> (-30.569, -91.8212) centre (-29.7181, -91.8212) ccw
  arc A239 (-30.569, -91.8212) -> (-28.8672, -91.8212) centre (-29.7181, -91.8212) ccw
  arc A240 (3.7211, -91.7954) -> (7.7089, -91.7954) centre (5.715, -91.7954) ccw
  arc A241 (7.7089, -91.7954) -> (3.7211, -91.7954) centre (5.715, -91.7954) ccw
  arc A242 (9.9441, -91.9224) -> (11.6459, -91.9224) centre (10.795, -91.9224) ccw
  arc A243 (11.6459, -91.9224) -> (9.9441, -91.9224) centre (10.795, -91.9224) ccw
  arc A244 (1.4859, -91.9224) -> (-0.2159, -91.9224) centre (0.635, -91.9224) ccw
  arc A245 (-0.2159, -91.9224) -> (1.4859, -91.9224) centre (0.635, -91.9224) ccw
  arc A246 (-155.2574, -122.1302) -> (-159.2452, -122.1302) centre (-157.2513, -122.1302) ccw
  arc A247 (-159.2452, -122.1302) -> (-155.2574, -122.1302) centre (-157.2513, -122.1302) ccw
  arc A248 (-151.3204, -122.2572) -> (-153.0222, -122.2572) centre (-152.1713, -122.2572) ccw
  arc A249 (-153.0222, -122.2572) -> (-151.3204, -122.2572) centre (-152.1713, -122.2572) ccw
  arc A250 (-161.4804, -122.2572) -> (-163.1822, -122.2572) centre (-162.3313, -122.2572) ccw
  arc A251 (-163.1822, -122.2572) -> (-161.4804, -122.2572) centre (-162.3313, -122.2572) ccw
  arc A252 (-112.598, -122.1302) -> (-116.5859, -122.1302) centre (-114.5919, -122.1302) ccw
  arc A253 (-116.5859, -122.1302) -> (-112.598, -122.1302) centre (-114.5919, -122.1302) ccw
  arc A254 (-108.661, -122.2572) -> (-110.3628, -122.2572) centre (-109.5119, -122.2572) ccw
  arc A255 (-110.3628, -122.2572) -> (-108.661, -122.2572) centre (-109.5119, -122.2572) ccw
  arc A256 (-118.8211, -122.2572) -> (-120.5229, -122.2572) centre (-119.672, -122.2572) ccw
  arc A257 (-120.5229, -122.2572) -> (-118.8211, -122.2572) centre (-119.672, -122.2572) ccw
  arc A258 (-82.598, -122.1302) -> (-86.5859, -122.1302) centre (-84.5919, -122.1302) ccw
  arc A259 (-86.5859, -122.1302) -> (-82.598, -122.1302) centre (-84.5919, -122.1302) ccw
  arc A260 (-78.661, -122.2572) -> (-80.3628, -122.2572) centre (-79.5119, -122.2572) ccw
  arc A261 (-80.3628, -122.2572) -> (-78.661, -122.2572) centre (-79.5119, -122.2572) ccw
  arc A262 (-90.5229, -122.2572) -> (-88.8211, -122.2572) centre (-89.672, -122.2572) ccw
  arc A263 (-88.8211, -122.2572) -> (-90.5229, -122.2572) centre (-89.672, -122.2572) ccw
  arc A264 (-52.598, -122.1302) -> (-56.5859, -122.1302) centre (-54.5919, -122.1302) ccw
  arc A265 (-56.5859, -122.1302) -> (-52.598, -122.1302) centre (-54.5919, -122.1302) ccw
  arc A266 (-48.661, -122.2572) -> (-50.3628, -122.2572) centre (-49.5119, -122.2572) ccw
  arc A267 (-50.3628, -122.2572) -> (-48.661, -122.2572) centre (-49.5119, -122.2572) ccw
  arc A268 (-60.5229, -122.2572) -> (-58.8211, -122.2572) centre (-59.672, -122.2572) ccw
  arc A269 (-58.8211, -122.2572) -> (-60.5229, -122.2572) centre (-59.672, -122.2572) ccw
  arc A270 (-22.598, -122.1302) -> (-26.5859, -122.1302) centre (-24.5919, -122.1302) ccw
  arc A271 (-26.5859, -122.1302) -> (-22.598, -122.1302) centre (-24.5919, -122.1302) ccw
  arc A272 (-20.3628, -122.2572) -> (-18.661, -122.2572) centre (-19.5119, -122.2572) ccw
  arc A273 (-18.661, -122.2572) -> (-20.3628, -122.2572) centre (-19.5119, -122.2572) ccw
  arc A274 (-30.5229, -122.2572) -> (-28.8211, -122.2572) centre (-29.672, -122.2572) ccw
  arc A275 (-28.8211, -122.2572) -> (-30.5229, -122.2572) centre (-29.672, -122.2572) ccw
  arc A276 (3.4141, -122.1302) -> (7.402, -122.1302) centre (5.4081, -122.1302) ccw
  line L31 (7.402, -122.1302) -> (7.402, -122.1302)
  arc A277 (7.402, -122.1302) -> (3.4141, -122.1302) centre (5.4081, -122.1302) ccw
  arc A278 (11.339, -122.2572) -> (9.6372, -122.2572) centre (10.4881, -122.2572) ccw
  arc A279 (9.6372, -122.2572) -> (11.339, -122.2572) centre (10.4881, -122.2572) ccw
  arc A280 (1.1789, -122.2572) -> (-0.5229, -122.2572) centre (0.328, -122.2572) ccw
  arc A281 (-0.5229, -122.2572) -> (1.1789, -122.2572) centre (0.328, -122.2572) ccw
  arc A282 (33.4141, -122.1302) -> (37.402, -122.1302) centre (35.4081, -122.1302) ccw
  arc A283 (37.402, -122.1302) -> (33.4141, -122.1302) centre (35.4081, -122.1302) ccw
  arc A284 (41.339, -122.2572) -> (39.6372, -122.2572) centre (40.4881, -122.2572) ccw
  arc A285 (39.6372, -122.2572) -> (41.339, -122.2572) centre (40.4881, -122.2572) ccw
  arc A286 (31.1789, -122.2572) -> (29.4771, -122.2572) centre (30.328, -122.2572) ccw
  arc A287 (29.4771, -122.2572) -> (31.1789, -122.2572) centre (30.328, -122.2572) ccw
  arc A288 (-168.9187, 33.9116) -> (-167.4186, 33.9116) centre (-168.1687, 33.9116) ccw
  arc A289 (-167.4186, 33.9116) -> (-168.9187, 33.9116) centre (-168.1687, 33.9116) ccw
  arc A290 (-168.8679, 26.8936) -> (-167.3678, 26.8936) centre (-168.1179, 26.8936) ccw
  arc A291 (-167.3678, 26.8936) -> (-168.8679, 26.8936) centre (-168.1179, 26.8936) ccw
  line L32 (-184.318, 18.453) -> (-184.318, 22.253)
  line L33 (-180.518, 18.453) -> (-184.318, 18.453)
  line L34 (-180.518, 22.253) -> (-180.518, 18.453)
  line L35 (-184.318, 22.253) -> (-180.518, 22.253)
  line L36 (-154.318, 22.253) -> (-150.518, 22.253)
  line L37 (-154.318, 18.453) -> (-154.318, 22.253)
  line L38 (-150.518, 18.453) -> (-154.318, 18.453)
  line L39 (-150.518, 22.253) -> (-150.518, 18.453)
  line L40 (-124.318, 22.253) -> (-120.518, 22.253)
  line L41 (-120.518, 18.453) -> (-124.318, 18.453)
  line L42 (-124.318, 18.453) -> (-124.318, 22.253)
  line L43 (-120.518, 22.253) -> (-120.518, 18.453)
  line L44 (-94.318, 22.253) -> (-90.518, 22.253)
  line L45 (-94.318, 18.453) -> (-94.318, 22.253)
  line L46 (-90.518, 18.453) -> (-94.318, 18.453)
  line L47 (-90.518, 22.253) -> (-90.518, 18.453)
  line L48 (-64.318, 22.253) -> (-60.518, 22.253)
  line L49 (-60.518, 22.253) -> (-60.518, 18.453)
  line L50 (-60.518, 18.453) -> (-64.318, 18.453)
  line L51 (-64.318, 18.453) -> (-64.318, 22.253)
  line L52 (-30.518, 22.253) -> (-30.518, 18.453)
  line L53 (-34.318, 18.453) -> (-34.318, 22.253)
  line L54 (-30.518, 18.453) -> (-34.318, 18.453)
  line L55 (-34.318, 22.253) -> (-30.518, 22.253)
  line L56 (-0.518, 22.253) -> (-0.518, 18.453)
  line L57 (-0.518, 18.453) -> (-4.318, 18.453)
  line L58 (-4.318, 18.453) -> (-4.318, 22.253)
  line L59 (-4.318, 22.253) -> (-0.518, 22.253)
  line L60 (29.482, 18.453) -> (25.682, 18.453)
  line L61 (25.682, 18.453) -> (25.682, 22.253)
  line L62 (25.682, 22.253) -> (29.482, 22.253)
  line L63 (29.482, 22.253) -> (29.482, 18.453)
  line L64 (-180.518, -11.547) -> (-184.318, -11.547)
  line L65 (-180.518, -7.747) -> (-180.518, -11.547)
  line L66 (-184.318, -11.547) -> (-184.318, -7.747)
  line L67 (-184.318, -7.747) -> (-180.518, -7.747)
  line L68 (-154.318, -7.747) -> (-150.518, -7.747)
  line L69 (-154.318, -11.547) -> (-154.318, -7.747)
  line L70 (-150.518, -7.747) -> (-150.518, -11.547)
  line L71 (-150.518, -11.547) -> (-154.318, -11.547)
  line L72 (-120.518, -7.747) -> (-120.518, -11.547)
  line L73 (-120.518, -11.547) -> (-124.318, -11.547)
  line L74 (-124.318, -11.547) -> (-124.318, -7.747)
  line L75 (-124.318, -7.747) -> (-120.518, -7.747)
  line L76 (-90.518, -11.547) -> (-94.318, -11.547)
  line L77 (-94.318, -11.547) -> (-94.318, -7.747)
  line L78 (-90.518, -7.747) -> (-90.518, -11.547)
  line L79 (-94.318, -7.747) -> (-90.518, -7.747)
  line L80 (-64.318, -11.547) -> (-64.318, -7.747)
  line L81 (-64.318, -7.747) -> (-60.518, -7.747)
  line L82 (-60.518, -11.547) -> (-64.318, -11.547)
  line L83 (-60.518, -7.747) -> (-60.518, -11.547)
  line L84 (-30.518, -11.547) -> (-34.318, -11.547)
  line L85 (-34.318, -11.547) -> (-34.318, -7.747)
  line L86 (-34.318, -7.747) -> (-30.518, -7.747)
  line L87 (-30.518, -7.747) -> (-30.518, -11.547)
  line L88 (13.833, -11.801) -> (10.033, -11.801)
  line L89 (10.033, -11.801) -> (10.033, -8.001)
  line L90 (13.833, -8.001) -> (13.833, -11.801)
  line L91 (10.033, -8.001) -> (13.833, -8.001)
  line L92 (52.9491, -12.055) -> (49.1491, -12.055)
  line L93 (49.1491, -12.055) -> (49.1491, -8.255)
  line L94 (49.1491, -8.255) -> (52.9491, -8.255)
  line L95 (52.9491, -8.255) -> (52.9491, -12.055)
  line L96 (-196.538, -36.3221) -> (-192.738, -36.3221)
  line L97 (-192.738, -36.3221) -> (-192.738, -40.1221)
  line L98 (-196.538, -40.1221) -> (-196.538, -36.3221)
  line L99 (-192.738, -40.1221) -> (-196.538, -40.1221)
  line L100 (-166.538, -40.1221) -> (-166.538, -36.3221)
  line L101 (-166.538, -36.3221) -> (-162.738, -36.3221)
  line L102 (-162.738, -36.3221) -> (-162.738, -40.1221)
  line L103 (-162.738, -40.1221) -> (-166.538, -40.1221)
  line L104 (-132.738, -36.3221) -> (-132.738, -40.1221)
  line L105 (-136.538, -36.3221) -> (-132.738, -36.3221)
  line L106 (-136.538, -40.1221) -> (-136.538, -36.3221)
  line L107 (-132.738, -40.1221) -> (-136.538, -40.1221)
  line L108 (-106.538, -36.3221) -> (-102.738, -36.3221)
  line L109 (-106.538, -40.1221) -> (-106.538, -36.3221)
  line L110 (-102.738, -36.3221) -> (-102.738, -40.1221)
  line L111 (-102.738, -40.1221) -> (-106.538, -40.1221)
  line L112 (-72.738, -40.1221) -> (-76.538, -40.1221)
  line L113 (-72.738, -36.3221) -> (-72.738, -40.1221)
  line L114 (-76.538, -40.1221) -> (-76.538, -36.3221)
  line L115 (-76.538, -36.3221) -> (-72.738, -36.3221)
  line L116 (-46.538, -36.3221) -> (-42.738, -36.3221)
  line L117 (-42.738, -40.1221) -> (-46.538, -40.1221)
  line L118 (-46.538, -40.1221) -> (-46.538, -36.3221)
  line L119 (-42.738, -36.3221) -> (-42.738, -40.1221)
  line L120 (-12.738, -40.1221) -> (-16.538, -40.1221)
  line L121 (-16.538, -36.3221) -> (-12.738, -36.3221)
  line L122 (-12.738, -36.3221) -> (-12.738, -40.1221)
  line L123 (-16.538, -40.1221) -> (-16.538, -36.3221)